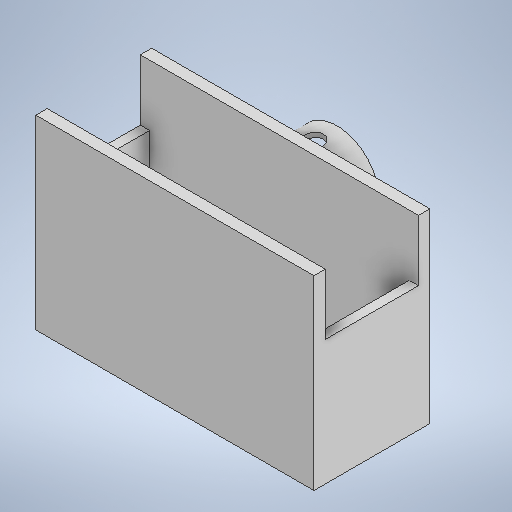
# Autodesk Inventor part: Attache servomoteur_bogie
Saved by Autodesk Inventor 2026.2 (Build 302298010, 298A)
## iProperties
Created: 2026-03-22
Part Number: Attache servomoteur_bogie
Material: Générique
Document SubType Name: Modeling
Designer: Genon
Density: 1 g/cm^3
Appearance: Par défaut
Author: Genon
Autodesk Inventor part; units mm, degrees
ref_plane "YZ Plane" through (0, 0, 0) normal (1, 0, 0) x (0, 1, 0)
ref_plane "XZ Plane" through (0, 0, 0) normal (0, 1, 0) x (-1, 0, 0)
ref_plane "XY Plane" through (0, 0, 0) normal (0, 0, 1) x (1, 0, 0)
sketch "Esquisse1" plane through (0, 0, 0) normal (0, 1, 0) x (-1, 0, 0)
  line L0 (0, 0) -> (0, 2.45)
  line L1 (0, 0) -> (2.45, 0) construction
  line L2 (0, 2.45) -> (28, 2.45)
  line L3 (28, 2.45) -> (28, 22.55)
  line L4 (28, 22.55) -> (-28, 22.55)
  line L5 (-28, 22.55) -> (-28, 2.45)
  line L6 (-28, 2.45) -> (0, 2.45)
  line L7 (0, 0) -> (30, 0)
  line L8 (30, 0) -> (30, 25)
  line L9 (30, 25) -> (-30, 25)
  line L10 (-30, 25) -> (-30, 0)
  line L11 (-30, 0) -> (0, 0)
  dimension "d0" = 2.45
  dimension "d1" = 90
  dimension "d2" = 28
  dimension "d3" = 20.1
  dimension "d4" = 56
  dimension "d5" = 30
  dimension "d6" = 25
  dimension "d7" = 60
  constraints: 24 end point, 6 perpendicular, 4 horizontal, 2 parallel, 1 point on line, 1 vertical
  measures "d0" distance of L0.start L0.end
  measures "d1" angle of L1 L0
  measures "d2" distance of L0.end L2.end
  measures "d3" distance of L2.end L3.end
  measures "d4" distance of L3.end L4.end
  measures "d5" distance of L0.start L7.end
  measures "d6" distance of L7.end L8.end
  measures "d7" distance of L8.end L9.end
extrude "Extrusion1" add sketch "Esquisse1" along normal blind 27
sketch "Esquisse2" plane through (30, 0, 0) normal (0, 0, -1) x (-1, 0, 0)
  line L0 (30, 0) -> (30, 27)
  line L1 (60, 27) -> (0, 27) projected
  line L2 (0, 0) -> (0, 27) projected
  line L3 (0, 13.5) -> (60, 13.5)
  line L4 (60, 0) -> (60, 27) projected
  circle A0 centre (30, 13.5) radius 8
  circle A1 centre (30, 13.5) radius 9
  dimension "d10" = 16
  dimension "d11" = 18
  constraints: 4 end point, 4 midpoint, 2 centre point, 1 coincident
  measures "d10" diameter of A0
  measures "d11" diameter of A1
extrude "Extrusion2" add sketch "Esquisse2" along normal blind 10 contours A1 L3 A0 L0 | L0 A0 L3 A1 | A1 L0 A0 L3 | L3 A0 L0 A1
sketch "Esquisse3" plane through (0, 0, 0) normal (0, 1, 0) x (-1, 0, 0)
  line L0 (-9, -10) -> (9, -10) projected
  line L1 (0, -10) -> (0, -5)
  point P0 (0, 0)
  dimension "d14" = 5
  constraints: 2 end point, 1 coincident, 1 midpoint, 1 vertical
  measures "d14" distance of L1.start L1.end
hole "Perçage1" at (0, 0, -5) direction (0, 1, 0) diameter 4 end through all
sketch "Esquisse7" plane through (0, 0, 0) normal (0, -1, 0) x (1, 0, 0)
  line L0 (-30, 0) -> (-30, 25) projected
  line L1 (30, 0) -> (-30, 0) projected
  line L2 (30, 25) -> (30, 0) projected
  line L3 (-30, 25) -> (30, 25) projected
  line L4 (28, 22.55) -> (-28, 22.55) projected
  line L5 (-28, 2.45) -> (28, 2.45) projected
  line L6 (-28, 22.55) -> (-28, 2.45) projected
  line L7 (28, 2.45) -> (28, 22.55) projected
  point P0 (0, 0)
extrude "Extrusion5" add sketch "Esquisse7" along normal blind 13.14
sketch "Esquisse11" plane through (0, -13.14, 0) normal (0, -1, 0) x (1, 0, 0)
  line L0 (28, 22.55) -> (28, 2.45) projected
  line L1 (-28, 22.55) -> (28, 22.55) projected
  line L2 (28, 2.45) -> (28, 22.55) projected
  line L3 (28, 22.55) -> (28, 2.45)
  line L4 (28, 22.55) -> (-28, 22.55) projected
  line L5 (28, 22.55) -> (22, 22.55)
  line L6 (22, 22.55) -> (22, 2.45)
  line L7 (22, 2.45) -> (28, 2.45)
  line L8 (-28, 22.55) -> (-22, 22.55)
  line L9 (-22, 22.55) -> (-22, 2.45)
  line L10 (-28, 2.45) -> (28, 2.45) projected
  line L11 (-22, 2.45) -> (-28, 2.45)
  line L12 (-28, 22.55) -> (-28, 2.45) projected
  line L13 (-28, 22.55) -> (-28, 2.45)
  point P0 (0, 0)
  dimension "d46" = 6
  dimension "d47" = 6
  constraints: 16 end point, 4 perpendicular, 2 point on line, 1 collinear, 1 vertical
  measures "d46" distance of L0.start L5.end
  measures "d47" distance of L1.start L8.end
extrude "Extrusion6" add sketch "Esquisse11" against normal blind 9 contours L0 L7 L6 L1 | L9 L10 L12 L1
sketch "Esquisse12" plane through (0, -4.14, 0) normal (0, 1, 0) x (1, 0, 0)
  line L0 (-22, -22.55) -> (-28, -22.55) projected
  line L1 (-28, -22.55) -> (-28, -13.5)
  line L2 (-28, -22.55) -> (-28, -2.45) projected
  line L3 (-28, -13.5) -> (-22, -13.5)
  line L4 (-22, -22.55) -> (-22, -2.45) projected
  line L5 (-22, -13.5) -> (-22, -11.5)
  line L6 (-22, -11.5) -> (-28, -11.5)
  line L7 (-28, -13.5) -> (-28, -11.5)
  line L8 (-28, -11.5) -> (-28, -13.5)
  line L9 (28, -2.45) -> (28, -22.55) projected
  line L10 (28, -22.55) -> (28, -13.5)
  line L11 (28, -13.5) -> (22, -13.5)
  line L12 (22, -13.5) -> (22, -11.5)
  line L13 (22, -22.55) -> (22, -2.45) projected
  line L14 (22, -11.5) -> (28, -11.5)
  line L15 (28, -11.5) -> (28, -13.5)
  line L16 (28, -13.5) -> (28, -11.5)
  point P0 (0, 0)
  dimension "d50" = 9.05
  dimension "d51" = 2
  dimension "d52" = 6
  constraints: 24 end point, 10 point on line, 5 perpendicular, 1 collinear, 1 horizontal
  measures "d50" distance of L0.end L1.end
  measures "d51" distance of L3.end L5.end
  measures "d52" distance of L10.end L11.end
extrude "Extrusion7" cut sketch "Esquisse12" against normal blind 2 contours L3 L2 L6 L4 | L9 L11 L12 L14
sketch "Esquisse13" plane through (0, -4.14, 0) normal (0, 1, 0) x (1, 0, 0)
  line L0 (-28, -22.55) -> (-28, -2.45) projected
  line L1 (-28, -22.55) -> (-28, -12.5)
  line L2 (-28, -2.45) -> (-22, -2.45) projected
  line L3 (-28, -12.5) -> (-25, -12.5)
  line L4 (-25, -12.5) -> (-25, -7.5)
  line L5 (-25, -12.5) -> (-25, -17.5)
  line L6 (28, -13.5) -> (28, -22.55) projected
  line L7 (28, -22.55) -> (28, -12.5)
  line L8 (28, -12.5) -> (25, -12.5)
  line L9 (25, -12.5) -> (25, -7.5)
  line L10 (25, -7.5) -> (25, -17.5)
  point P0 (0, 0)
  dimension "d55" = 10.05
  dimension "d56" = 3
  dimension "d57" = 5
  dimension "d58" = 5
  dimension "d59" = 3
  dimension "d60" = 5
  dimension "d61" = 10
  constraints: 16 end point, 5 perpendicular, 4 coincident, 2 vertical, 1 point on line
  measures "d55" distance of L0.start L1.end
  measures "d56" distance of L1.end L3.end
  measures "d57" distance of L3.end L4.end
  measures "d58" distance of L3.end L5.end
  measures "d59" distance of L7.end L8.end
  measures "d60" distance of L8.end L9.end
  measures "d61" distance of L9.end L10.end
hole "Perçage3" at (-25, -4.14, 17.5) at (-25, -4.14, 7.5) at (25, -4.14, 17.5) at (25, -4.14, 7.5) direction (0, -1, 0) diameter 3.242 depth 11.8 tip angle 118 thread size "M4x0.7" class "6H" standard "ISO Metric profile"
sketch "Esquisse14" plane through (30, 27, 25) normal (1, 0, 0) x (0, 0, -1)
  line L0 (0, -40.14) -> (0, 0) projected
  line L1 (0, 0) -> (2.45, 0)
  line L2 (0, 0) -> (25, 0) projected
  line L3 (2.45, 0) -> (2.45, -13.14)
  line L4 (2.45, -31.14) -> (2.45, -40.14) projected
  line L5 (2.45, -13.14) -> (22.55, -13.14)
  line L6 (22.55, -13.14) -> (22.55, 0)
  line L7 (2.45, 0) -> (22.55, 0)
  line L8 (25, -40.14) -> (25, 0) projected
  point P0 (25, -27)
  dimension "d69" = 2.45
  dimension "d70" = 13.14
  dimension "d71" = 20.1
  constraints: 10 end point, 3 perpendicular, 2 point on line, 1 collinear
  measures "d69" distance of L0.end L1.end
  measures "d70" distance of L1.end L3.end
  measures "d71" distance of L3.end L5.end
extrude "Extrusion8" cut sketch "Esquisse14" against normal through all
